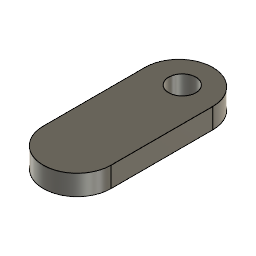
ACOPLE_SERVO (Autodesk Fusion 360 design; units mm, degrees)
Autodesk Fusion 360 part; units mm, degrees
sketch "Boceto1" plane through (0, 0, 0) normal (0, 0, 1) x (1, 0, 0)
  line L0 (-5, -7.5) -> (-5, 7.5)
  circle A0 centre (0, 8) radius 2
  line L1 (-6, 0) -> (7, 0) construction
  line L2 (0, 8) -> (0, -7) construction
  line L3 (5, -7.5) -> (5, 7.5)
  arc A1 (5, 7.5) -> (-5, 7.5) centre (0, 7.5) ccw
  arc A2 (-5, -7.5) -> (5, -7.5) centre (0, -7.5) ccw
  point P0 (-5, 0)
  point P1 (5, 0)
  dimension "d7" = 15
  dimension "d11" = 4
  dimension "d13" = 5
  dimension "d15" = 15
  dimension "d16" = 5
  constraint midpoint L0 P0
  constraint vertical L0
  constraint perpendicular L1 L2
  constraint coincident P0 L1
  constraint midpoint L3 P1
  constraint coincident L1 P1
  constraint perpendicular L1 L3
  constraint tangent L0 A1
  constraint tangent L0 A2
  constraint coincident A0.centre L2.start
  measures "d7" distance of L0.start L0.end
  measures "d11" diameter of A0
  measures "d13" distance of L0 L2
  measures "d15" distance of L3.start L3.end
  measures "d16" distance of L2 L3
extrude "Extruir1" add sketch "Boceto1" along normal blind 3
